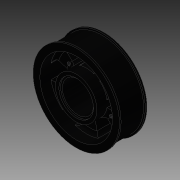
# Autodesk Inventor part: Wheel V1
Saved by Autodesk Inventor 2013 (Build 170138000, 138)
## iProperties
Created: 2013-04-01
Part Number: Wheel V1
Material: Generic
Document SubType Name: Modeling
Designer: mvarma
Density: 1 g/cm^3
Author: mvarma
Autodesk Inventor part; units mm, degrees
ref_plane "YZ Plane" through (0, 0, 0) normal (1, 0, 0) x (0, 1, 0)
ref_plane "XZ Plane" through (0, 0, 0) normal (0, 1, 0) x (-1, 0, 0)
ref_plane "XY Plane" through (0, 0, 0) normal (0, 0, 1) x (1, 0, 0)
sketch "Sketch1" plane through (0, 0, 0) normal (0, 0, 1) x (1, 0, 0)
  circle A0 centre (0, 0) radius 14.2875
  circle A1 centre (0, 0) radius 19.05
  circle A2 centre (0, 0) radius 38.1
  circle A3 centre (0, 0) radius 33.3375
  line L0 (-4.123175, 18.598439) -> (-7.215556, 32.547268)
  line L1 (4.123175, 18.598439) -> (7.215556, 32.547268)
  line L2 (0, 33.3375) -> (0, 19.05) construction
  line L3 (-4.123175, 18.598439) -> (0, 0) construction
  line L4 (4.123175, 18.598439) -> (0, 0) construction
  line L5 (0, 19.05) -> (0, 14.2875) construction
  line L6 (0, 14.2875) -> (0, 0) construction
  circle A4 centre (0, 0) radius 15.875
  dimension "d3" = 28.575
  dimension "d0" = 76.2
  dimension "d2" = 66.675
  dimension "d4" = 38.1
  dimension "d6" = 12.5
  dimension "d7" = 12.5
  dimension "d69" = 31.75
  constraints: 14 end point, 6 coincident, 6 point on circle, 4 centre point, 3 vertical, 2 collinear, 1 vertical alignment, 2 other
  measures "d0" diameter of A2
  measures "d2" diameter of A3
  measures "d4" diameter of A1
  measures "d6" angle of L0 L2
  measures "d7" angle of L2 L1
  measures "d69" diameter of A4
sketch "Sketch1 outline for Extrusion7" plane through (0, 0, 0) normal (0, 0, 1) x (1, 0, 0)
  circle A0 centre (0, 0) radius 38.1
  circle A1 centre (0, 0) radius 33.3375
  circle A2 centre (0, 0) radius 19.05
  circle A3 centre (0, 0) radius 14.2875
extrude "Extrusion7" add sketch "Sketch1 outline for Extrusion7" along normal blind 25.4
sketch "Sketch1 outline for Extrusion13" plane through (0, 0, 0) normal (0, 0, 1) x (1, 0, 0)
  circle A0 centre (0, 0) radius 15.875
  circle A1 centre (0, 0) radius 14.2875
extrude "Extrusion13" cut sketch "Sketch1 outline for Extrusion13" along normal blind 1.5875
sketch "Sketch1 outline for Extrusion9" plane through (0, 0, 0) normal (0, 0, 1) x (1, 0, 0)
  arc A0 (7.215556, 32.547268) -> (-7.215556, 32.547268) centre (0, 0) ccw
  line L0 (4.123175, 18.598439) -> (7.215556, 32.547268)
  arc A1 (-4.123175, 18.598439) -> (4.123175, 18.598439) centre (0, 0) cw
  line L1 (-7.215556, 32.547268) -> (-4.123175, 18.598439)
extrude "Extrusion9" add sketch "Sketch1 outline for Extrusion9" along normal blind 12.7
fillet "Fillet3" radius 3.175 6 edges at (7.2156, 32.5473, 6.35) (-7.2156, 32.5473, 6.35) (-4.1232, 18.5984, 6.35) (4.1232, 18.5984, 6.35) (0, 19.05, 12.7) (0, 33.3375, 12.7)
pattern_circular "Circular Pattern3" count 6 over 360 about axis through (0, 0, -10) along (0, 0, 1) of "Extrusion9", "Fillet3"
sketch "Sketch3" plane through (0, 0, 0) normal (0, 0, -1) x (-1, 0, 0)
  circle A0 centre (0, 0) radius 38.1
  circle A1 centre (0, 0) radius 39.6875
  arc A2 (-10.601497, 31.606916) -> (10.601497, 31.606916) centre (0, 0) ccw
  line L0 (0, 22.225) -> (0, 0) construction
  point P0 (-19.247415, 11.1125)
  point P1 (-19.247415, -11.1125)
  point P2 (0, -22.225)
  point P3 (19.247415, -11.1125)
  point P4 (19.247415, 11.1125)
  dimension "d51" = 22.225
  dimension "d54" = 360
  dimension "d63" = 79.375
  constraints: 2 coincident, 2 end point, 1 centre point, 1 vertical, 7 other
  measures "d51" distance of A0.centre L0.start
  measures "d63" diameter of A1
sketch "Sketch3 outline for Extrusion10" plane through (0, 0, 0) normal (0, 0, -1) x (-1, 0, 0)
  circle A0 centre (0, 0) radius 39.6875
  circle A1 centre (0, 0) radius 38.1
extrude "Extrusion10" add sketch "Sketch3 outline for Extrusion10" against normal blind 1.5875
sketch "Sketch4" plane through (0, 0, 25.4) normal (0, 0, 1) x (1, 0, 0)
  circle A0 centre (0, 0) radius 38.1 projected
  circle A1 centre (0, 0) radius 39.6875 projected
sketch "Sketch4 outline for Extrusion11" plane through (0, 0, 25.4) normal (0, 0, 1) x (1, 0, 0)
  circle A0 centre (0, 0) radius 39.6875
  circle A1 centre (0, 0) radius 38.1
extrude "Extrusion11" add sketch "Sketch4 outline for Extrusion11" against normal blind 1.5875
hole "Hole1" at (0, 22.225, 0) at (19.247415, 11.1125, 0) at (19.247415, -11.1125, 0) at (0, -22.225, 0) at (-19.247415, -11.1125, 0) at (-19.247415, 11.1125, 0) direction (0, 0, 1) diameter 3.302 depth 12.7 tip angle 118 thread size "8-32 UNC" class "2B" standard "ANSI Unified Screw Threads"
sketch "Sketch5" plane through (0, 0, 25.4) normal (0, 0, 1) x (1, 0, 0)
  circle A0 centre (0, 0) radius 14.2875 projected
  circle A1 centre (0, 0) radius 19.05 projected
  circle A2 centre (0, 0) radius 15.875
  dimension "d64" = 31.75
  constraints: 1 centre point, 1 coincident
  measures "d64" diameter of A2
sketch "Sketch5 outline for Extrusion12" plane through (0, 0, 25.4) normal (0, 0, 1) x (1, 0, 0)
  circle A0 centre (0, 0) radius 15.875
  circle A1 centre (0, 0) radius 14.2875
extrude "Extrusion12" cut sketch "Sketch5 outline for Extrusion12" against normal blind 1.5875
equation "\"d6\" = d7"
body "Solid2"
